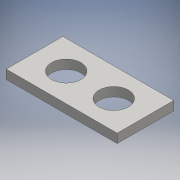
# Autodesk Inventor part: bearing support
Saved by Autodesk Inventor 2016 SP1 (Build 200210100, 210)
## iProperties
Created: 2016-05-25
Part Number: bearing support
Material: Generic
Document SubType Name: Modeling
Designer: ubik
Density: 1 g/cm^3
Appearance: Default
Author: ubik
Autodesk Inventor part; units mm, degrees
ref_plane "YZ Plane" through (0, 0, 0) normal (1, 0, 0) x (0, 1, 0)
ref_plane "XZ Plane" through (0, 0, 0) normal (0, 1, 0) x (-1, 0, 0)
ref_plane "XY Plane" through (0, 0, 0) normal (0, 0, 1) x (1, 0, 0)
sketch "Sketch1" plane through (0, 0, 0) normal (0, 0, 1) x (1, 0, 0)
  circle A0 centre (-21, 0) radius 13
  circle A1 centre (21, 0) radius 13
  line L0 (-49, 25) -> (49, 25)
  line L1 (49, 25) -> (49, -25)
  line L2 (49, -25) -> (-49, -25)
  line L3 (-49, -25) -> (-49, 25)
  point P0 (0, 0)
  dimension "d0" = 26
  dimension "d1" = 26
  dimension "d2" = 42
  dimension "d3" = 21
  dimension "d4" = 25
  dimension "d5" = 50
  dimension "d6" = 15
  dimension "d7" = 15
  constraints: 8 end point, 2 centre point, 2 parallel, 1 horizontal, 1 perpendicular
  measures "d0" diameter of A0
  measures "d1" diameter of A1
  measures "d2" distance of A1.centre A0.centre
  measures "d3" distance of point (0, 0) A0.centre
  measures "d4" distance from line of point (0, 0) L0
  measures "d5" distance of L2.end L0.start
  measures "d6" distance edge to line of A0 L3
  measures "d7" distance edge to line of A1 L1
extrude "Extrusion1" add sketch "Sketch1" along normal blind 8
equation "\"d3\" = 0.5 * d2"
equation "\"d7\" = d6"
body "Solid1"
